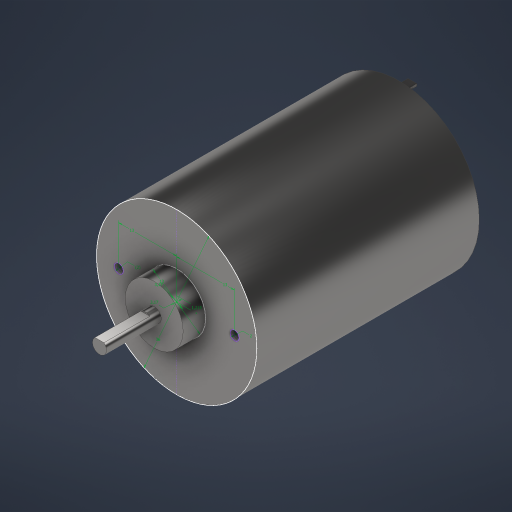
# Autodesk Inventor part: Motor
Saved by Autodesk Inventor 2023 (Build 270158000, 158)
## iProperties
Created: 2022-06-18
Part Number: Motor
Material: Stainless Steel
Document SubType Name: Modeling
Designer: Levi
Density: 8 g/cm^3
Appearance: Semi-Polished
Author: Levi
Autodesk Inventor part; units mm, degrees
ref_plane "YZ Plane" through (0, 0, 0) normal (1, 0, 0) x (0, 1, 0)
ref_plane "XZ Plane" through (0, 0, 0) normal (0, 1, 0) x (-1, 0, 0)
ref_plane "XY Plane" through (0, 0, 0) normal (0, 0, 1) x (1, 0, 0)
sketch "Sketch1" plane through (0, 0, 0) normal (0, 0, 1) x (1, 0, 0)
  circle A0 centre (0, 0) radius 18
  circle A1 centre (0, 0) radius 6.5
  arc A2 (-1.0178, 1.215) -> (1.0178, 1.215) centre (0, 0) ccw
  line L0 (-1.585, 0) -> (1.585, 0)
  line L1 (-1.0178, 1.215) -> (1.0178, 1.215)
  circle A3 centre (13, 0) radius 1
  line L2 (0, -18) -> (0, 18) construction
  circle A4 centre (-13, 0) radius 1
  circle A5 centre (0, 0) radius 1.585
  point P0 (1.0178, 1.215)
  point P1 (-1.0178, 1.215)
  dimension "d0" = 36
  dimension "d1" = 13
  dimension "d2" = 3.17
  dimension "d3" = 1.215
  dimension "d4" = 13
  dimension "d5" = 2
  dimension "d6" = 13
  dimension "d7" = 2
  dimension "d36" = 3.17
  constraints: 9 coincident, 6 centre point, 6 end point, 6 point on circle, 2 symmetric about line, 1 horizontal, 1 midpoint, 1 parallel, 1 point on line, 1 vertical, 1 other
  measures "d0" diameter of A0
  measures "d1" diameter of A1
  measures "d2" diameter of A2
  measures "d3" distance between parallel lines of L0 L1
  measures "d4" distance of point (0, 0) point (13, 0)
  measures "d5" diameter of A3
  measures "d6" distance of A0.centre A4.centre
  measures "d7" diameter of A4
  measures "d36" diameter of A5
extrude "Extrusion1" add sketch "Sketch1" along normal blind 17.3 and the other way blind 51.5 contours L1 A2 L0 | L0 A2
extrude "Extrusion2" add sketch "Sketch1" along normal blind 5 and the other way blind 51 contours A1 | A5 L1
extrude "Extrusion3" add sketch "Sketch1" against normal blind 50 contours A0 | A3 | A4
hole "Hole2" at (0, 0, 0) at (13, 0, 0) at (-13, 0, 0) direction (0, 0, -1) diameter 2 depth 8 tip angle 118
thread "Thread1" size "M2x0.4" class "6H" standard "ANSI Metric M Profile" full length
thread "Thread2" size "M2x0.4" class "6H" standard "ANSI Metric M Profile" full length
extrude "Extrusion4" add sketch "Sketch1" along normal blind 7 and the other way blind 51.5 contours L1 A2 L0 | A5 L1 | L0 A2
sketch "Sketch2" plane through (0, 0, -50) normal (0, 0, -1) x (-1, 0, 0)
  line L0 (-1, 16.45) -> (1, 16.45)
  line L1 (1, 16.45) -> (1, 15.95)
  line L2 (1, 15.95) -> (-1, 15.95)
  line L3 (-1, 15.95) -> (-1, 16.45)
  line L4 (-1, 16.45) -> (1, 15.95) construction
  line L5 (1, 16.45) -> (-1, 15.95) construction
  line L6 (0, 0) -> (0, 18) construction
  circle A0 centre (0, 0) radius 18 projected
  line L7 (0, 0) -> (-18, 0) construction
  line L8 (-1, -16.45) -> (1, -16.45)
  line L9 (1, -16.45) -> (1, -15.95)
  line L10 (1, -15.95) -> (-1, -15.95)
  line L11 (-1, -15.95) -> (-1, -16.45)
  line L12 (-1, -16.45) -> (1, -15.95) construction
  line L13 (1, -16.45) -> (-1, -15.95) construction
  point P0 (0, 16.2)
  point P1 (0, -16.2)
  dimension "d41" = 2
  dimension "d42" = 0.5
  constraints: 28 end point, 5 symmetric about line, 2 horizontal, 2 midpoint, 2 parallel, 2 point on circle, 1 perpendicular, 1 point on line, 1 vertical
  measures "d41" distance of L1.end L2.end
  measures "d42" distance of L0.end L1.end
extrude "Extrusion5" add sketch "Sketch2" along normal blind 3 contours L0 L1 L2 L3 | L11 L10 L9 L8
body "Solid1"
